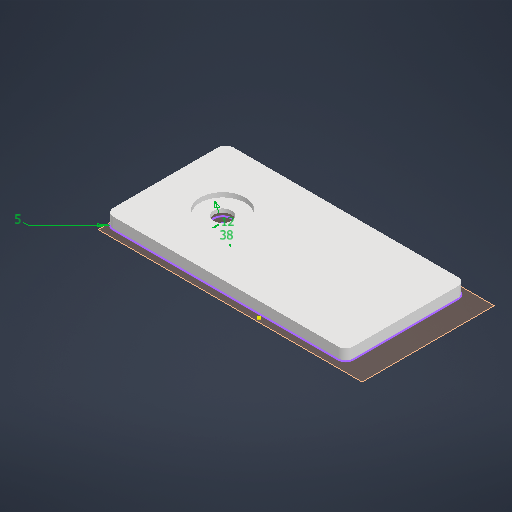
# Autodesk Inventor part: BaseTop
Saved by Autodesk Inventor 2026.1 (Build 301233020, 233B)
## iProperties
Created: 2025-10-21
Part Number: BaseTop
Material: Generic
Document SubType Name: Modeling
Designer: Nathan
Density: 1 g/cm^3
Appearance: Default
Author: Nathan
Autodesk Inventor part; units mm, degrees
ref_plane "YZ Plane" through (0, 0, 0) normal (1, 0, 0) x (0, 1, 0)
ref_plane "XZ Plane" through (0, 0, 0) normal (0, 1, 0) x (-1, 0, 0)
ref_plane "XY Plane" through (0, 0, 0) normal (0, 0, 1) x (1, 0, 0)
ref_plane "Work Plane1" through (-24.4516, 95.9016, -42.078) normal (0, 1, 0) x (-1, 0, 0)
sketch "BaseTop" plane through (-24.4516, 95.9016, -42.078) normal (0, 1, 0) x (-1, 0, 0)
  line L0 (75, 40) -> (-75, 40)
  line L1 (-80, 35) -> (-80, -35)
  line L2 (-75, -40) -> (75, -40)
  line L3 (80, -35) -> (80, 35)
  circle A0 centre (42, 0) radius 6
  arc A1 (80, 35) -> (75, 40) centre (75, 35) ccw
  arc A2 (75, -40) -> (80, -35) centre (75, -35) ccw
  arc A3 (-80, -35) -> (-75, -40) centre (-75, -35) ccw
  arc A4 (-75, 40) -> (-80, 35) centre (-75, 35) ccw
  circle A5 centre (42, 0) radius 19
  point P0 (-24.4516, 42.078)
  dimension "d1" = 12
  dimension "d2" = 5
  dimension "d15" = 38
  constraints: 8 end point, 8 point on circle, 8 tangent, 6 centre point, 3 equal radius, 2 parallel, 1 coincident, 1 horizontal, 1 perpendicular
  measures "d1" diameter of A0
  measures "d2" radius of A1
  measures "d15" diameter of A5
extrude "Extrusion1" add sketch "BaseTop" along normal blind 7.5 contours A1 L3 A2 L2 A3 L1 A4 L0 | A0 | A5
extrude "Extrusion6" cut sketch "BaseTop" along normal blind 2 contours A0 | A5
sketch "Sketch6" plane through (-24.4516, 103.4016, -42.078) normal (0, 1, 0) x (1, 0, 0)
  circle A0 centre (-42, 0) radius 15
  point P0 (24.4516, -42.078)
  dimension "d20" = 30
  constraints: 1 centre point
  measures "d20" diameter of A0
extrude "Extrusion7" cut sketch "Sketch6" against normal blind 3
extrude "Extrusion8" cut sketch "BaseTop" along normal through all contours A0
body "Solid3"
